Autodesk Inventor part; units mm, degrees
(part 2 of 2)
extrude "Vysunutí3" cut sketch "Náčrt6" against normal blind 0.1 contours S0 S1 L18 L19 L20 S2 S3 | S8 S9 S10 S11 L24 L25 S12 S13 S14 L26 L27 S15 S16 | S21 L29 L30 S22 S23 S24 S25 S26 S27 S28 S29 S30 L31 L32 S31 S32 S33 S34 S35 S36 S37 | L33 L34 L35 L36 | L37 L38 L39 L40 | S38 S39 S40 S41 L41 S42 S43 S44 S45 S46 L42 L43 L44 S47 S48 L45 L46 | L48 L49 S53 S54 S55 L50 L51 L52 L53 L54 S56 S57 L55 | S58 S59 S60 S61 L56 L57 S62 S63 S64 L58 L59 S65 S66 | L61 L62 S71 S72 S73 S74 S75 S76 S77 L63 L64 L65 | S82 S83 L67 L68 L69 L70 L71 S84 S85 | L73 L74 L75 L76 L77 L78 L79 L80 | S90 L81 L82 S91 S92 S93 S94 S95 S96 S97 S98 L83 L84 S99 S100 S101 S102 S103 S104 S105 | S106 L85 L86 L87 L88 L89 L90 L91 L92 L93 L94 L95 S107 S108 S109 L96 L97 S110 | S111 S112 S113 S114 S115 S116 L98 S117 S118 S119 L99 L100 S120 S121 S122 L101 L102 L103 | S127 L105 L106 S128 S129 S130 S131 S132 S133 S134 S135 S136 L107 L108 S137 S138 S139 S140 S141 S142 S143 | S144 L109 L110 L111 L112 L113 L114 L115 L116 L117 L118 L119 S145 S146 S147 L120 L121 S148 | L122 L123 S149 S150 S151 L124 L125 L126 L127 L128 S152 S153 L129 | L130 L131 L132 L133 L134 L135 L136 L137 | L138 L139 L140 L141 L142 L143 L144 L145 L146 L147 L148 L149 L150 | S154 S155 S156 S157 S158 S159 L151 S160 S161 S162 L152 L153 S163 S164 S165 L154 L155 L156 | S170 S171 S172 S173 S174 L158 L159 S175 S176 S177 S178 S179 L160 L161 S180 S181 | L162 L163 S182 S183 S184 L164 L165 L166 L167 L168 S185 S186 L169 | L170 L171 L172 L173 | L174 L175 L176 L177 | L178 L179 S187 S188 S189 L180 L181 L182 L183 L184 S190 S191 L185 | S192 S193 S194 S195 L186 L187 S196 S197 S198 L188 L189 S199 S200 | L191 L192 S205 S206 S207 S208 S209 S210 S211 L193 L194 L195 | S216 S217 L197 L198 L199 L200 L201 S218 S219 | L203 L204 L205 L206 L207 L208 L209 L210 | L211 L212 L213 L214 L215 L216 L217 L218 L219 L220 L221 L222 | S224 S225 S226 S227 | L223 L224 S232 S233 S234 L225 L226 L227 S235 S236 S237 L228 L229 L230 | L231 L232 S238 S239 S240 S241 S242 S243 S244 L233 L234 L235 | S249 S250 S251 S252 L237 L238 S253 S254 S255 L239 L240 S256 S257 | L242 L243 L244 L245 L246 L247 L248 L249 L250 L251 L252 L253
ref_plane "Pracovní rovina3" through (-32, 0, -27.5) normal (0, 0, -1) x (-1, 0, 0)
